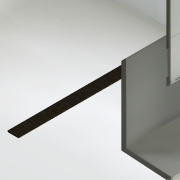
# Autodesk Inventor part: back_plate_gantry
Saved by Autodesk Inventor 2016 SP2 (Build 200236200, 236)
## iProperties
Created: 2017-09-11
Part Number: back_plate_gantry
Material: Generic
Document SubType Name: Modeling
Designer: Admin
Density: 1 g/cm^3
Appearance: Default
Mass: 3060 g
Surface Area: 4626 cm^2
Volume: 3060 cm^3
Author: Admin
Autodesk Inventor part; units mm, degrees
ref_plane "YZ Plane" through (0, 0, 0) normal (1, 0, 0) x (0, 1, 0)
ref_plane "XZ Plane" through (0, 0, 0) normal (0, 1, 0) x (-1, 0, 0)
ref_plane "XY Plane" through (0, 0, 0) normal (0, 0, 1) x (1, 0, 0)
sketch "Sketch1" plane through (0, 0, 0) normal (0, 0, 1) x (1, 0, 0)
  line L0 (230, 290) -> (0, 290) projected
  line L1 (0, -1410) -> (230, -1410) projected
  line L2 (0, -1410) -> (120, -1410)
  line L3 (120, -1410) -> (120, 290)
  line L4 (120, 290) -> (0, 290)
  line L5 (0, 290) -> (0, -1410)
  point P0 (0, 0)
  dimension "d0" = 120
  constraints: 8 end point, 2 parallel, 1 horizontal, 1 perpendicular, 1 point on line
  measures "d0" distance between parallel lines of L3 L5
extrude "Extrusion1" add sketch "Sketch1" along normal blind 15
body "Solid1"
